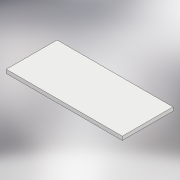
# Autodesk Inventor part: back
Saved by Autodesk Inventor 2017 (Build 210142000, 142)
## iProperties
Created: 2017-03-04
Part Number: back
Material: Acrylic
Document SubType Name: Modeling
Designer: dpgai
Density: 1.188 g/cm^3
Appearance: White
Author: dpgai
Autodesk Inventor part; units mm, degrees
ref_plane "YZ Plane" through (0, 0, 0) normal (1, 0, 0) x (0, 1, 0)
ref_plane "XZ Plane" through (0, 0, 0) normal (0, 1, 0) x (-1, 0, 0)
ref_plane "XY Plane" through (0, 0, 0) normal (0, 0, 1) x (1, 0, 0)
sketch "Sketch1" plane through (0, 0, 0) normal (0, 0, 1) x (1, 0, 0)
  line L0 (0, 0) -> (100, 0)
  line L1 (100, 0) -> (100, 43.764)
  line L2 (100, 43.764) -> (0, 43.764)
  line L3 (0, 43.764) -> (0, 0)
  dimension "d0" = 100
  dimension "d1" = 43.764
  constraints: 8 end point, 2 parallel, 1 horizontal, 1 perpendicular
  measures "d0" distance of L2.end L1.end
  measures "d1" distance of L1.end L0.end
extrude "Extrusion1" add sketch "Sketch1" along normal blind 3.175
sketch "Sketch2" plane through (0, 0, 0) normal (-1, 0, 0) x (0, 0, 1)
  line L0 (3.175, 0) -> (3.175, 43.764) projected
  line L1 (3.175, 43.764) -> (0, 44.3238)
  line L2 (3.175, 43.764) -> (21.1062, 43.764) construction
  line L3 (3.175, 43.764) -> (0, 43.764)
  line L4 (0, 43.764) -> (0, 44.3238)
  point P0 (0, 0)
  dimension "d4" = 170
  constraints: 8 end point, 2 horizontal, 1 perpendicular
  measures "d4" angle of L2 L1
extrude "Extrusion2" add sketch "Sketch2" against normal blind 100
body "Solid1"
